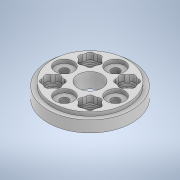
# Autodesk Inventor part: Inner_support_stand
Saved by Autodesk Inventor 2020.4 (Build 244396000, 396)
## iProperties
Created: 2021-09-25
Part Number: Inner_support_stand
Material: アルミニウム 2014-T4
Document SubType Name: Modeling
Designer: Masato Kubotera
Density: 2.8 g/cm^3
Appearance: 滑らか - 淡い灰色
Mass: 5.51581 g
Surface Area: 21.3058 cm^2
Volume: 1.96993 cm^3
Author: Masato Kubotera
Autodesk Inventor part; units mm, degrees
ref_plane "YZ Plane" through (0, 0, 0) normal (1, 0, 0) x (0, 1, 0)
ref_plane "XZ Plane" through (0, 0, 0) normal (0, 1, 0) x (-1, 0, 0)
ref_plane "XY Plane" through (0, 0, 0) normal (0, 0, 1) x (1, 0, 0)
derived "Inner_flange.ipt"
sketch "スケッチ1" plane through (0, 0, 0) normal (0, 0, 1) x (1, 0, 0)
  circle A0 centre (0, 0) radius 13.95
  line L0 (0, 13.95) -> (0, -13.95) construction
  circle A1 centre (0, 8.5) radius 1.35
  circle A2 centre (-8.5, 0) radius 1.35
  circle A3 centre (0, -8.5) radius 1.35
  circle A4 centre (8.5, 0) radius 1.35
  circle A5 centre (0, 0) radius 5 construction
  circle A6 centre (0, 0) radius 5.01
  circle A7 centre (-6.173, 6.173) radius 2.25
  line L1 (-9.8641, 9.8641) -> (9.8641, -9.8641) construction
  circle A8 centre (-6.173, 6.173) radius 1.55
  line L2 (-9.2514, 5.3482) -> (-8.9797, 6.3624) construction
  line L3 (-8.4266, 8.4266) -> (-7.4124, 8.6983) construction
  line L4 (-5.3482, 9.2514) -> (-4.6057, 8.509) construction
  line L5 (-3.0947, 6.9979) -> (-3.3664, 5.9837) construction
  line L6 (-3.9195, 3.9195) -> (-4.9337, 3.6478) construction
  line L7 (-6.9979, 3.0947) -> (-7.7404, 3.8371) construction
  circle A9 centre (0, 0) radius 12.45
  arc A10 (-7.4124, 8.6983) -> (-8.6983, 7.4124) centre (-7.6841, 7.6841) ccw
  arc A11 (-8.9797, 6.3624) -> (-8.509, 4.6057) centre (-8.2372, 5.62) ccw
  arc A12 (-7.7404, 3.8371) -> (-5.9837, 3.3664) centre (-6.7261, 4.1089) ccw
  arc A13 (-4.9337, 3.6478) -> (-3.6478, 4.9337) centre (-4.662, 4.662) ccw
  arc A14 (-3.3664, 5.9837) -> (-3.8371, 7.7404) centre (-4.1089, 6.7261) ccw
  arc A15 (-4.6057, 8.509) -> (-6.3624, 8.9797) centre (-5.62, 8.2372) ccw
  line L8 (-6.3624, 8.9797) -> (-5.3482, 9.2514) construction
  line L9 (-7.4124, 8.6983) -> (-6.3624, 8.9797)
  line L10 (-4.6057, 8.509) -> (-3.8371, 7.7404)
  line L11 (-3.8371, 7.7404) -> (-3.0947, 6.9979) construction
  line L12 (-3.3664, 5.9837) -> (-3.6478, 4.9337)
  line L13 (-3.6478, 4.9337) -> (-3.9195, 3.9195) construction
  line L14 (-4.9337, 3.6478) -> (-5.9837, 3.3664)
  line L15 (-5.9837, 3.3664) -> (-6.9979, 3.0947) construction
  line L16 (-7.7404, 3.8371) -> (-8.509, 4.6057)
  line L17 (-8.509, 4.6057) -> (-9.2514, 5.3482) construction
  line L18 (-8.9797, 6.3624) -> (-8.6983, 7.4124)
  line L19 (-8.6983, 7.4124) -> (-8.4266, 8.4266) construction
  circle A16 centre (-8.5, 0) radius 3.05
  line L20 (-8.6983, -7.4124) -> (-8.9797, -6.3624)
  circle A17 centre (-6.173, -6.173) radius 2.25
  circle A18 centre (-6.173, -6.173) radius 1.55
  circle A19 centre (0, -8.5) radius 3.05
  arc A20 (-3.8371, -7.7404) -> (-3.3664, -5.9837) centre (-4.1089, -6.7261) ccw
  line L21 (-3.6478, -4.9337) -> (-3.3664, -5.9837)
  arc A21 (-3.6478, -4.9337) -> (-4.9337, -3.6478) centre (-4.662, -4.662) ccw
  line L22 (-5.9837, -3.3664) -> (-4.9337, -3.6478)
  arc A22 (-5.9837, -3.3664) -> (-7.7404, -3.8371) centre (-6.7261, -4.1089) ccw
  line L23 (-8.509, -4.6057) -> (-7.7404, -3.8371)
  arc A23 (-8.509, -4.6057) -> (-8.9797, -6.3624) centre (-8.2372, -5.62) ccw
  arc A24 (-8.6983, -7.4124) -> (-7.4124, -8.6983) centre (-7.6841, -7.6841) ccw
  line L24 (-6.3624, -8.9797) -> (-7.4124, -8.6983)
  arc A25 (-6.3624, -8.9797) -> (-4.6057, -8.509) centre (-5.62, -8.2372) ccw
  line L25 (-3.8371, -7.7404) -> (-4.6057, -8.509)
  line L26 (7.4124, -8.6983) -> (6.3624, -8.9797)
  circle A26 centre (6.173, -6.173) radius 2.25
  circle A27 centre (6.173, -6.173) radius 1.55
  circle A28 centre (8.5, 0) radius 3.05
  arc A29 (7.7404, -3.8371) -> (5.9837, -3.3664) centre (6.7261, -4.1089) ccw
  line L27 (4.9337, -3.6478) -> (5.9837, -3.3664)
  arc A30 (4.9337, -3.6478) -> (3.6478, -4.9337) centre (4.662, -4.662) ccw
  line L28 (3.3664, -5.9837) -> (3.6478, -4.9337)
  arc A31 (3.3664, -5.9837) -> (3.8371, -7.7404) centre (4.1089, -6.7261) ccw
  line L29 (4.6057, -8.509) -> (3.8371, -7.7404)
  arc A32 (4.6057, -8.509) -> (6.3624, -8.9797) centre (5.62, -8.2372) ccw
  arc A33 (7.4124, -8.6983) -> (8.6983, -7.4124) centre (7.6841, -7.6841) ccw
  line L30 (8.9797, -6.3624) -> (8.6983, -7.4124)
  arc A34 (8.9797, -6.3624) -> (8.509, -4.6057) centre (8.2372, -5.62) ccw
  line L31 (7.7404, -3.8371) -> (8.509, -4.6057)
  line L32 (8.6983, 7.4124) -> (8.9797, 6.3624)
  circle A35 centre (6.173, 6.173) radius 2.25
  circle A36 centre (6.173, 6.173) radius 1.55
  circle A37 centre (0, 8.5) radius 3.05
  arc A38 (3.8371, 7.7404) -> (3.3664, 5.9837) centre (4.1089, 6.7261) ccw
  line L33 (3.6478, 4.9337) -> (3.3664, 5.9837)
  arc A39 (3.6478, 4.9337) -> (4.9337, 3.6478) centre (4.662, 4.662) ccw
  line L34 (5.9837, 3.3664) -> (4.9337, 3.6478)
  arc A40 (5.9837, 3.3664) -> (7.7404, 3.8371) centre (6.7261, 4.1089) ccw
  line L35 (8.509, 4.6057) -> (7.7404, 3.8371)
  arc A41 (8.509, 4.6057) -> (8.9797, 6.3624) centre (8.2372, 5.62) ccw
  arc A42 (8.6983, 7.4124) -> (7.4124, 8.6983) centre (7.6841, 7.6841) ccw
  line L36 (6.3624, 8.9797) -> (7.4124, 8.6983)
  arc A43 (6.3624, 8.9797) -> (4.6057, 8.509) centre (5.62, 8.2372) ccw
  line L37 (3.8371, 7.7404) -> (4.6057, 8.509)
  line L38 (-8.8035, 8.8035) -> (-3.5426, 3.5426) construction
  circle A44 centre (0, 0) radius 4
  point P0 (-9.2514, 5.3482)
  point P1 (-6.9979, 3.0947)
  point P2 (-3.9195, 3.9195)
  point P3 (-3.0947, 6.9979)
  point P4 (-3.0947, -6.9979)
  point P5 (-3.9195, -3.9195)
  point P6 (-6.9979, -3.0947)
  point P7 (-9.2514, -5.3482)
  point P8 (-8.4266, -8.4266)
  point P9 (-5.3482, -9.2514)
  point P10 (6.9979, -3.0947)
  point P11 (3.9195, -3.9195)
  point P12 (3.0947, -6.9979)
  point P13 (5.3482, -9.2514)
  point P14 (8.4266, -8.4266)
  point P15 (9.2514, -5.3482)
  point P16 (3.0947, 6.9979)
  point P17 (3.9195, 3.9195)
  point P18 (6.9979, 3.0947)
  point P19 (9.2514, 5.3482)
  point P20 (8.4266, 8.4266)
  point P21 (5.3482, 9.2514)
  point P22 (-9.2318, 8.3532)
  point P23 (-9.2318, -8.3532)
  point P24 (-8.3532, -9.2318)
  point P25 (8.3532, -9.2318)
  point P26 (9.2318, -8.3532)
  point P27 (9.2318, 8.3532)
  point P28 (8.3532, 9.2318)
  point P29 (-8.3532, 9.2318)
  point P30 (-6.173, 6.173)
  dimension "d37" = 24.9
  dimension "d3" = 4.5
  dimension "d4" = 45
  dimension "d6" = 10
  dimension "d26" = 3.1
  dimension "d38" = 1.05
  dimension "d41" = 360
  dimension "d43" = 5.52
  dimension "d44" = 6.1
  dimension "d47" = 360
  dimension "d50" = 8
  measures "d3" diameter of A7
  measures "d4" angle of L1 L0
  measures "d6" diameter of A5
  measures "d26" diameter of A8
  measures "d38" radius of A10
  measures "d43" distance between parallel lines of L12 L18
  measures "d44" diameter of A16
  measures "d50" diameter of A44
extrude "押し出し1" add sketch "スケッチ1" along normal blind 5 contours A6 | A9
extrude "押し出し2" add sketch "スケッチ1" along normal blind 3.75 contours A0
extrude "押し出し3" add sketch "スケッチ1" along normal blind 2.8 contours L9 A15 L10 A14 L12 A13 L14 A12 L16 A11 L18 A10 | L20 A23 L23 A22 L22 A21 L21 A20 L25 A25 L24 A24 | L26 A32 L29 A31 L28 A30 L27 A29 L31 A34 L30 A33 | L32 A41 L35 A40 L34 A39 L33 A38 L37 A43 L36 A42
extrude "押し出し4" add sketch "スケッチ1" along normal blind 2 contours A7 | A17 | A26 | A35
extrude "押し出し5" add sketch "スケッチ1" along normal blind 3.75 contours A16 | A19 | A28 | A37
equation "\"d34\" = d18"
equation "\"d18\" = 3.75"
